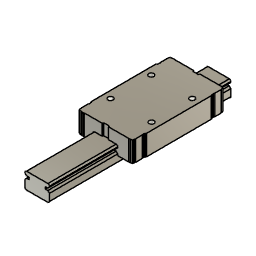
Wózek_prowadnica (Autodesk Fusion 360 design; units mm, degrees)
Autodesk Fusion 360 part; units mm, degrees
sketch "Szkic2" plane through (0, 0, 0) normal (0, 0, 1) x (1, 0, 0)
  line L0 (0.5477, 0.4589) -> (0.7, 0.3)
  line L1 (0.7, 0.3) -> (1.5, 0.1)
  line L2 (1.5, 0.1) -> (2.2904, 0.0655)
  line L3 (2.2904, 0.0655) -> (12.1473, 0.0943)
  line L4 (12.1473, 0.0943) -> (12.2508, 0.226)
  line L5 (12.2508, 0.226) -> (12.2979, 0.6305)
  line L6 (12.2979, 0.6305) -> (14.9884, 0.6384)
  line L7 (14.9884, 0.6384) -> (15.1105, 0.1602)
  line L8 (15.1105, 0.1602) -> (15.2422, 0.0849)
  line L9 (15.2422, 0.0849) -> (23.9813, 0.0755)
  line L10 (23.9813, 0.0755) -> (24.1318, -0.0185)
  line L11 (24.1318, -0.0185) -> (24.8468, -0.0193)
  line L12 (24.8468, -0.0193) -> (25.1383, 0.0473)
  line L13 (25.1383, 0.0473) -> (25.477, 0.0285)
  line L14 (25.477, 0.0285) -> (25.9944, 0.132)
  line L15 (25.9944, 0.132) -> (26.5172, 0.2365)
  line L16 (26.5172, 0.2365) -> (26.7093, 0.386)
  line L17 (26.7093, 0.386) -> (26.7658, 1.1103)
  line L18 (26.7658, 1.1103) -> (26.7846, 1.3737)
  line L19 (26.7846, 1.3737) -> (26.7093, 1.4583)
  line L20 (26.7093, 1.4583) -> (26.7991, 1.5382)
  line L21 (26.7991, 1.5382) -> (26.7991, 3.8)
  line L22 (26.7991, 3.8) -> (26.7752, 5.033)
  line L23 (26.7752, 5.033) -> (26.6905, 5.2399)
  line L24 (26.6905, 5.2399) -> (26.5964, 5.3905)
  line L25 (26.5964, 5.3905) -> (26.7469, 5.7009)
  line L26 (26.7469, 5.7009) -> (26.7187, 6.3217)
  line L27 (26.7187, 6.3217) -> (26.794, 6.4628)
  line L28 (26.794, 6.4628) -> (26.9182, 6.4584)
  line L29 (26.9182, 6.4584) -> (27.0302, 6.4999)
  line L30 (27.0302, 6.4999) -> (27.0298, 6.7378)
  line L31 (27.0298, 6.7378) -> (26.9182, 38.6182)
  line L32 (26.9182, 38.6182) -> (26.7385, 38.7234)
  line L33 (26.7385, 38.7234) -> (26.4901, 38.7638)
  line L34 (26.4901, 38.7638) -> (26.4901, 39.5761)
  line L35 (26.4901, 39.5761) -> (26.4001, 39.7061)
  line L36 (26.4001, 39.7061) -> (26.3026, 39.7711)
  line L37 (26.3026, 39.7711) -> (26.4526, 40.0485)
  line L38 (26.4526, 40.0485) -> (26.4776, 40.3735)
  line L39 (26.4776, 40.3735) -> (26.4951, 41.2983)
  line L40 (26.4951, 41.2983) -> (26.4968, 42.3691)
  line L41 (26.4968, 42.3691) -> (26.5013, 43.3724)
  line L42 (26.5013, 43.3724) -> (26.4887, 43.8502)
  line L43 (26.4887, 43.8502) -> (26.3606, 44.6632)
  line L44 (26.3606, 44.6632) -> (26.2, 44.8)
  line L45 (26.2, 44.8) -> (24.8739, 44.975)
  line L46 (24.8739, 44.975) -> (23.8326, 45.0084)
  line L47 (23.8326, 45.0084) -> (23.6823, 44.9193)
  line L48 (23.6823, 44.9193) -> (15, 44.9193)
  line L49 (15, 44.9193) -> (14.7953, 44.8414)
  line L50 (14.7953, 44.8414) -> (14.7, 44.4)
  line L51 (14.7, 44.4) -> (14.6673, 44.3458)
  line L52 (14.6673, 44.3458) -> (14, 44.3458)
  line L53 (14, 44.3458) -> (13.9156, 44.4237)
  line L54 (13.9156, 44.4237) -> (12.6, 44.4237)
  line L55 (12.6, 44.4237) -> (12.5736, 44.3458)
  line L56 (12.5736, 44.3458) -> (12.0446, 44.3402)
  line L57 (12.0446, 44.3402) -> (11.9444, 44.8024)
  line L58 (11.9444, 44.8024) -> (11.8, 44.9)
  line L59 (11.8, 44.9) -> (1.6, 44.9)
  line L60 (1.6, 44.9) -> (0.2956, 44.5713)
  line L61 (0.2956, 44.5713) -> (0.2, 43.7)
  line L62 (0.2, 43.7) -> (0.1898, 43.5829)
  line L63 (0.1898, 43.5829) -> (0.084, 43.5105)
  line L64 (0.084, 43.5105) -> (0.084, 40.4)
  line L65 (0.084, 40.4) -> (0.1938, 39.763)
  line L66 (0.1938, 39.763) -> (0.2522, 39.6776)
  line L67 (0.2522, 39.6776) -> (0.1741, 39.4042)
  line L68 (0.1741, 39.4042) -> (0.183, 38.7697)
  line L69 (0.183, 38.7697) -> (-0.0903, 38.7047)
  line L70 (-0.0903, 38.7047) -> (-0.1887, 38.5749)
  line L71 (-0.1887, 38.5749) -> (-0.0982, 38.3979)
  line L72 (-0.0982, 38.3979) -> (0, 6.6)
  line L73 (0, 6.6) -> (0.0316, 6.3256)
  line L74 (0.0316, 6.3256) -> (0.4567, 6.1485)
  line L75 (0.4567, 6.1485) -> (0.4583, 5.6223)
  line L76 (0.4583, 5.6223) -> (0.4876, 5.3675)
  line L77 (0.4876, 5.3675) -> (0.5427, 5.2629)
  line L78 (0.5427, 5.2629) -> (0.4061, 4.9289)
  line L79 (0.4061, 4.9289) -> (0.3657, 3.1467)
  line L80 (0.3657, 3.1467) -> (0.3282, 1.4919)
  line L81 (0.3282, 1.4919) -> (0.4744, 1.4321)
  line L82 (0.4744, 1.4321) -> (0.4219, 1.3038)
  line L83 (0.4219, 1.3038) -> (0.4716, 1.178)
  line L84 (0.4716, 1.178) -> (0.5322, 0.6214)
  line L85 (0.5322, 0.6214) -> (0.5477, 0.4589)
  circle A0 centre (23.448, 32.6514) radius 1.8526
  circle A1 centre (3.4408, 32.6002) radius 1.8346
  circle A2 centre (23.5356, 12.6463) radius 1.8379
  circle A3 centre (3.4921, 12.5855) radius 1.8455
  circle A4 centre (23.448, 32.6514) radius 1.5
  circle A5 centre (3.4408, 32.6002) radius 1.5
  circle A6 centre (23.5356, 12.6463) radius 1.5
  circle A7 centre (3.4921, 12.5855) radius 1.5
  dimension "d3" = 3
  dimension "d4" = 3
  dimension "d5" = 3
  dimension "d6" = 3
  constraint parallel L3 L6
  constraint parallel L9 L11
  constraint parallel L14 L15
  constraint perpendicular L19 L20
  constraint vertical L21
  constraint vertical L34
  constraint horizontal L48
  constraint parallel L48 L52
  constraint parallel L52 L54
  constraint horizontal L59
  constraint vertical L64
  constraint perpendicular L63 L66
  constraint parallel L72 L75
  constraint parallel L73 L76
  constraint parallel L79 L80
  constraint perpendicular L78 L81
  constraint perpendicular L81 L82
  constraint concentric A0 A4
  constraint concentric A1 A5
  constraint concentric A2 A6
  constraint concentric A3 A7
  measures "d3" diameter of A4
  measures "d4" diameter of A5
  measures "d5" diameter of A6
  measures "d6" diameter of A7
extrude "Wyciągnięcie proste1" add sketch "Szkic2" along normal blind 10 contours L0 L1 L2 L3 L4 L5 L6 L7 L8 L9 L10 L11 L12 L13 L14 L15 L16 L17 L18 L19 L20 L21 L22 L23 L24 L25 L26 L27 L28 L29 L30 L31 L32 L33 L34 L35 L36 L37 L38 L39 L40 L41 L42 L43 L44 L45 L46 L47 L48 L49 L50 L51 L52 L53 L54 L55 L56 L57 L58 L59 L60 L61 L62 L63 L64 L65 L66 L67 L68 L69 L70 L71 L72 L73 L74 L75 L76 L77 L78 L79 L80 L81 L82 L83 L84 L85 | A0 | A1 | A2 | A3 | A4 | A5 | A6 | A7 makes body 1
extrude "Wyciągnięcie proste2" cut sketch "Szkic2" along normal blind 6 contours A4 | A5 | A6 | A7 bodies 1
thread "Gwint1" "ISO Metric profile 3.0 M3x0.5 6H" major diameter 3.086 minor diameter 2.529 pitch 0.5 angle 60 resizes the face on face at (4.9902, 12.5108, 4) on bodies 1
thread "Gwint2" "ISO Metric profile 3.0 M3x0.5 6H" major diameter 3.086 minor diameter 2.529 pitch 0.5 angle 60 resizes the face on face at (25.0282, 12.7956, 4) on bodies 1
thread "Gwint3" "ISO Metric profile 3.0 M3x0.5 6H" major diameter 3.086 minor diameter 2.529 pitch 0.5 angle 60 resizes the face on face at (4.8504, 33.1132, 4) on bodies 1
thread "Gwint4" "ISO Metric profile 3.0 M3x0.5 6H" major diameter 3.086 minor diameter 2.529 pitch 0.5 angle 60 resizes the face on face at (24.8576, 33.1645, 4) on bodies 1
sketch "Szkic1" plane through (0, 0, 0) normal (0, 0, 1) x (1, 0, 0) in component "prowadnica_szyna v3"
  line L0 (0.75, 0) -> (11.25, 0)
  line L1 (11.25, 8) -> (0.75, 8)
  line L2 (6, 0) -> (6, 8)
  line L3 (12, 0.75) -> (12, 1.3964)
  line L4 (11.3964, 2) -> (10.5, 2)
  line L5 (10.5, 2) -> (10.5, 3)
  line L6 (10.5, 3) -> (11.3964, 3)
  line L7 (12, 0.75) -> (12, 1.3964)
  line L8 (12, 3.6036) -> (12, 7.25)
  line L9 (11.5732, 1.9268) -> (11.9268, 1.5732)
  line L10 (11.5732, 3.0732) -> (11.9268, 3.4268)
  arc A0 (11.5732, 1.9268) -> (11.3964, 2) centre (11.3964, 1.75) ccw
  arc A1 (12, 1.3964) -> (11.9268, 1.5732) centre (11.75, 1.3964) ccw
  arc A2 (11.3964, 3) -> (11.5732, 3.0732) centre (11.3964, 3.25) ccw
  arc A3 (11.9268, 3.4268) -> (12, 3.6036) centre (11.75, 3.6036) ccw
  arc A4 (11.25, 0) -> (12, 0.75) centre (11.25, 0.75) ccw
  arc A5 (12, 7.25) -> (11.25, 8) centre (11.25, 7.25) ccw
  line L11 (0.6036, 2) -> (1.5, 2)
  line L12 (0.4268, 1.9268) -> (0.0732, 1.5732)
  arc A6 (0, 0.75) -> (0.75, 0) centre (0.75, 0.75) ccw
  line L13 (0, 0.75) -> (0, 1.3964)
  line L14 (1.5, 2) -> (1.5, 3)
  line L15 (1.5, 3) -> (0.6036, 3)
  line L16 (0.4268, 3.0732) -> (0.0732, 3.4268)
  arc A7 (0.4268, 3.0732) -> (0.6036, 3) centre (0.6036, 3.25) ccw
  arc A8 (0, 3.6036) -> (0.0732, 3.4268) centre (0.25, 3.6036) ccw
  line L17 (0, 3.6036) -> (0, 7.25)
  arc A9 (0.75, 8) -> (0, 7.25) centre (0.75, 7.25) ccw
  arc A10 (0.0732, 1.5732) -> (0, 1.3964) centre (0.25, 1.3964) ccw
  arc A11 (0.6036, 2) -> (0.4268, 1.9268) centre (0.6036, 1.75) ccw
  line L18 (0, 7.25) -> (0, 3.6036)
  point P0 (12, 3)
  point P1 (11.5, 2)
  point P2 (12, 1.5)
  point P3 (11.5, 3)
  point P4 (12, 3.5)
  dimension "d3_1" = 1
  dimension "d6_1" = 0.5
  dimension "d7_1" = 0.5
  dimension "d8_1" = 0.25
  dimension "d9" = 0.75
  constraint horizontal L0
  constraint vertical L7
  constraint horizontal L1
  constraint vertical L18
  constraint perpendicular L4 L7
  constraint perpendicular L4 L5
  constraint coincident P0 L7
  constraint perpendicular L6 L7
  constraint collinear L7 L8
  constraint coincident P0 L6
  constraint coincident P0 L8
  constraint coincident P1 L9
  constraint coincident L4 P1
  constraint tangent L9 A0
  constraint tangent L4 A0
  constraint coincident P2 L9
  constraint coincident L3 P2
  constraint tangent L9 A1
  constraint tangent L3 A1
  constraint equal A0 A1
  constraint coincident P3 L10
  constraint coincident L6 P3
  constraint tangent L10 A2
  constraint tangent L6 A2
  constraint equal A0 A2
  constraint coincident P4 L10
  constraint coincident L8 P4
  constraint tangent L10 A3
  constraint tangent L8 A3
  constraint equal A0 A3
  constraint coincident L0 L2.start
  constraint tangent L0 A4
  constraint tangent L3 A4
  constraint coincident L1 L2.end
  constraint tangent L1 A5
  constraint tangent L8 A5
  constraint equal A4 A5
  constraint symmetric L2 L4.end L11.end
  constraint symmetric L2 L5.end L14.end
  constraint symmetric L2 L9.start L12.start
  constraint symmetric L2 L4.start L11.start
  constraint symmetric L2 A0 A11
  constraint symmetric L2 L9.end L12.end
  constraint symmetric L2 L3.end L13.end
  constraint symmetric L2 A1 A10
  constraint symmetric L2 L10.start L16.start
  constraint symmetric L2 L6.end L15.end
  constraint symmetric L2 A2 A7
  constraint symmetric L2 L10.end L16.end
  constraint symmetric L2 L8.start A8.start
  constraint symmetric L2 A3 A8
  constraint symmetric L2 L0.end L0.start
  constraint symmetric L2 L3.start A6.start
  constraint symmetric L2 A4 A6
  constraint symmetric L2 L1.start L1.end
  constraint symmetric L2 L8.end L17.end
  constraint symmetric L2 A5 A9
  measures "d3_1" distance of L4.end L5.end
  measures "d6_1" distance of P0 P3
  measures "d7_1" distance of P0 P4
  measures "d8_1" radius of A0
  measures "d9" radius of A4
extrude "Wyciągnięcie proste1'" add sketch "Szkic1" along normal blind 80 separate body makes body 2 in component "prowadnica_szyna v3"
sketch "Szkic2 (2)" plane through (0, 0, 80) normal (0, 0, 1) x (-1, 0, 0) in component "prowadnica_szyna v3"
  arc A0 (-11.5732, -1.9268) -> (-11.3964, -2) centre (-11.3964, -1.75) ccw
  line L0 (-11.3964, -2) -> (-10.5, -2)
  line L1 (-10.5, -2) -> (-10.5, -3)
  line L2 (-10.5, -3) -> (-11.3964, -3)
  arc A1 (-11.3964, -3) -> (-11.5732, -3.0732) centre (-11.3964, -3.25) ccw
  line L3 (-11.5732, -3.0732) -> (-11.9268, -3.4268)
  arc A2 (-11.9268, -3.4268) -> (-12, -3.6036) centre (-11.75, -3.6036) ccw
  line L4 (-12, -3.6036) -> (-12, -7.25)
  arc A3 (-12, -7.25) -> (-11.25, -8) centre (-11.25, -7.25) ccw
  line L5 (-11.25, -8) -> (-0.75, -8)
  arc A4 (-0.75, -8) -> (0, -7.25) centre (-0.75, -7.25) ccw
  line L6 (0, -7.25) -> (0, -3.6036)
  arc A5 (0, -3.6036) -> (-0.0732, -3.4268) centre (-0.25, -3.6036) ccw
  line L7 (-0.0732, -3.4268) -> (-0.4268, -3.0732)
  arc A6 (-0.4268, -3.0732) -> (-0.6036, -3) centre (-0.6036, -3.25) ccw
  line L8 (-0.6036, -3) -> (-1.5, -3)
  line L9 (-1.5, -3) -> (-1.5, -2)
  line L10 (-1.5, -2) -> (-0.6036, -2)
  arc A7 (-0.6036, -2) -> (-0.4268, -1.9268) centre (-0.6036, -1.75) ccw
  line L11 (-0.4268, -1.9268) -> (-0.0732, -1.5732)
  arc A8 (-0.0732, -1.5732) -> (0, -1.3964) centre (-0.25, -1.3964) ccw
  line L12 (0, -1.3964) -> (0, -0.75)
  arc A9 (0, -0.75) -> (-0.75, 0) centre (-0.75, -0.75) ccw
  line L13 (-0.75, 0) -> (-11.25, 0)
  arc A10 (-11.25, 0) -> (-12, -0.75) centre (-11.25, -0.75) ccw
  line L14 (-12, -0.75) -> (-12, -1.3964)
  arc A11 (-12, -1.3964) -> (-11.9268, -1.5732) centre (-11.75, -1.3964) ccw
  line L15 (-11.9268, -1.5732) -> (-11.5732, -1.9268)
  line L16 (0, -3.6036) -> (-2, -3.6036)
  line L17 (-2, -3.6036) -> (-2, -1.6787)
  line L18 (-1.5, -2) -> (-2, -2)
  line L19 (-1.5, -3) -> (-2, -3)
  line L20 (-6, 0) -> (-6, -8.8189)
  line L21 (-10.5, -3) -> (-10, -3)
  line L22 (-10.5, -2) -> (-10, -2)
  line L23 (-10, -3.6036) -> (-10, -1.6787)
  constraint coincident L6.end A5.start
  constraint perpendicular L6 L16
  constraint perpendicular L10 L17
  constraint coincident L9.end L10.start
  constraint coincident L17 L18.end
  constraint perpendicular L17 L18
  constraint coincident L8.end L9.start
  constraint coincident L17 L19.end
  constraint perpendicular L17 L19
  constraint midpoint L13 L20.start
  constraint perpendicular L13 L20
  constraint symmetric L16.end L20 L23.start
  constraint symmetric L17.end L20 L23.end
  constraint symmetric L9.end L20 L0.end
  constraint symmetric L18.end L20 L22.end
  constraint symmetric L8.end L20 L1.end
  constraint symmetric L19.end L20 L21.end
extrude "Wyciągnięcie proste2'" cut sketch "Szkic2 (2)" against normal blind 104 contours L1 L21 L22 L23 | L9 L17 L18 L19 bodies 2 in component "prowadnica_szyna v3"
sketch "Szkic3" plane through (0, 0, 80) normal (0, 0, 1) x (-1, 0, 0) in component "prowadnica_szyna v3"
  line L0 (-10, -3) -> (-11.3964, -3)
  arc A0 (-11.3964, -3) -> (-11.5732, -3.0732) centre (-11.3964, -3.25) ccw
  line L1 (-11.5732, -3.0732) -> (-11.9268, -3.4268)
  arc A1 (-11.9268, -3.4268) -> (-12, -3.6036) centre (-11.75, -3.6036) ccw
  line L2 (-12, -3.6036) -> (-12, -7.25)
  arc A2 (-12, -7.25) -> (-11.25, -8) centre (-11.25, -7.25) ccw
  line L3 (-11.25, -8) -> (-0.75, -8)
  arc A3 (-0.75, -8) -> (0, -7.25) centre (-0.75, -7.25) ccw
  line L4 (0, -7.25) -> (0, -3.6036)
  arc A4 (0, -3.6036) -> (-0.0732, -3.4268) centre (-0.25, -3.6036) ccw
  line L5 (-0.0732, -3.4268) -> (-0.4268, -3.0732)
  arc A5 (-0.4268, -3.0732) -> (-0.6036, -3) centre (-0.6036, -3.25) ccw
  line L6 (-0.6036, -3) -> (-2, -3)
  line L7 (-2, -3) -> (-2, -2)
  line L8 (-2, -2) -> (-0.6036, -2)
  arc A6 (-0.6036, -2) -> (-0.4268, -1.9268) centre (-0.6036, -1.75) ccw
  line L9 (-0.4268, -1.9268) -> (-0.0732, -1.5732)
  arc A7 (-0.0732, -1.5732) -> (0, -1.3964) centre (-0.25, -1.3964) ccw
  line L10 (0, -1.3964) -> (0, -0.75)
  arc A8 (0, -0.75) -> (-0.75, 0) centre (-0.75, -0.75) ccw
  line L11 (-0.75, 0) -> (-11.25, 0)
  arc A9 (-11.25, 0) -> (-12, -0.75) centre (-11.25, -0.75) ccw
  line L12 (-12, -0.75) -> (-12, -1.3964)
  arc A10 (-12, -1.3964) -> (-11.9268, -1.5732) centre (-11.75, -1.3964) ccw
  line L13 (-11.9268, -1.5732) -> (-11.5732, -1.9268)
  arc A11 (-11.5732, -1.9268) -> (-11.3964, -2) centre (-11.3964, -1.75) ccw
  line L14 (-11.3964, -2) -> (-10, -2)
  line L15 (-10, -2) -> (-10, -3)
  line L16 (0, -3) -> (-0.9, -3)
  line L17 (-0.9357, -2) -> (0, -2)
  line L18 (0, -2) -> (0, -1.2)
  line L19 (0, -3.8) -> (0, -4.6)
  line L20 (-0.8, -3) -> (-1.6, -3)
  line L21 (-0.8, -3) -> (0, -3.8)
  line L22 (-2, -2.5) -> (0.6, -2.5)
  line L23 (-0.8, -2) -> (0, -1.2)
  line L24 (-6, 0) -> (-6, -4)
  line L25 (-11.2, -3) -> (-12, -3.8)
  line L26 (-11.2, -2) -> (-12, -1.2)
  dimension "d14" = 0.8
  dimension "d15" = 0.8
  constraint coincident L6 L16.end
  constraint coincident L8 L17.start
  constraint perpendicular L7 L17
  constraint coincident L10 L18.end
  constraint perpendicular L17 L18
  constraint coincident L4 L19.end
  constraint perpendicular L16 L19
  constraint coincident L6 L20.end
  constraint coincident L16.start L20
  constraint coincident L16.start L19
  constraint midpoint L7 L22.start
  constraint perpendicular L7 L22
  constraint symmetric L20.start L22 L23.start
  constraint symmetric L19.start L22 L18.end
  constraint midpoint L11 L24.start
  constraint perpendicular L11 L24
  constraint symmetric L20.start L24 L25.start
  constraint symmetric L19.start L24 L25.end
  constraint symmetric L23.start L24 L26.start
  constraint symmetric L18.end L24 L26.end
  measures "d14" distance of L16.start L20.start
  measures "d15" distance of L16.start L19.start
extrude "Wyciągnięcie proste3" cut sketch "Szkic3" against normal blind 97 contours L0 A0 L1 A1 L2 L25 | L12 A10 L13 A11 L14 L26 | L4 A4 L5 A5 L6 L16 L21 | L8 A6 L9 A7 L10 L17 L18 L23 bodies 2 in component "prowadnica_szyna v3"
extrude "Wyciągnięcie proste4" cut 1 faces at (4.6667, 6.3333, 80) along direction (0, 0, -1) blind 25 on bodies 2 bodies 2 in component "prowadnica_szyna v3"
move_body "Przesuń1" bodies 1 to x (-0.999981, -0.006176, 0) y (-0.006176, 0.999981, 0) z (0, 0, -1) at (27.0406, 0.0835, 10)
sketch "Szkic3 (2)" plane through (0, -23.685, 0) normal (0, -1, 0) x (1, 0, 0)
  line L0 (0.8, 28.315) -> (0, 27.515)
  line L1 (0, 27.515) -> (0, 24.065)
  arc A0 (0, 24.065) -> (0.75, 23.315) centre (0.75, 24.065) ccw
  line L2 (0.75, 23.315) -> (11.25, 23.315)
  arc A1 (11.25, 23.315) -> (12, 24.065) centre (11.25, 24.065) ccw
  line L3 (12, 24.065) -> (12, 27.515)
  line L4 (12, 27.515) -> (11.2, 28.315)
  line L5 (11.2, 28.315) -> (10, 28.315)
  line L6 (10, 28.315) -> (10, 29.315)
  line L7 (10, 29.315) -> (11.2, 29.315)
  line L8 (11.2, 29.315) -> (12, 30.115)
  line L9 (12, 30.115) -> (12, 30.565)
  arc A2 (12, 30.565) -> (11.25, 31.315) centre (11.25, 30.565) ccw
  line L10 (11.25, 31.315) -> (0.75, 31.315)
  arc A3 (0.75, 31.315) -> (0, 30.565) centre (0.75, 30.565) ccw
  line L11 (0, 30.565) -> (0, 30.115)
  line L12 (0, 30.115) -> (0.8, 29.315)
  line L13 (0.8, 29.315) -> (2, 29.315)
  line L14 (2, 29.315) -> (2, 28.315)
  line L15 (2, 28.315) -> (0.8, 28.315)
  line L16 (6, 23.315) -> (6, 26.815)
  line L17 (0, 26.815) -> (12, 26.815)
  dimension "d20" = 3.5
  constraint midpoint L2 L16.start
  constraint perpendicular L2 L16
  constraint coincident L1 L17.start
  constraint coincident L3 L17.end
  constraint perpendicular L3 L17
  measures "d20" distance of L16.start L16.end
sketch "Szkic4" plane through (0, 0, 0) normal (0, 0, -1) x (1, 0, 0)
  line L0 (26.5046, -0.7016) -> (26.4901, -0.539)
  line L1 (26.4901, -0.539) -> (26.3388, -0.3792)
  line L2 (26.3388, -0.3792) -> (25.54, -0.1742)
  line L3 (25.54, -0.1742) -> (24.7499, -0.1349)
  line L4 (24.7499, -0.1349) -> (14.8929, -0.1028)
  line L5 (14.8929, -0.1028) -> (14.7886, -0.2339)
  line L6 (14.7886, -0.2339) -> (14.7391, -0.6381)
  line L7 (14.7391, -0.6381) -> (12.0486, -0.6293)
  line L8 (12.0486, -0.6293) -> (11.9294, -0.1504)
  line L9 (11.9294, -0.1504) -> (11.7982, -0.0743)
  line L10 (11.7982, -0.0743) -> (3.0593, -0.0109)
  line L11 (3.0593, -0.0109) -> (2.9094, 0.0841)
  line L12 (2.9094, 0.0841) -> (2.1945, 0.0893)
  line L13 (2.1945, 0.0893) -> (1.9025, 0.0244)
  line L14 (1.9025, 0.0244) -> (1.5639, 0.0454)
  line L15 (1.5639, 0.0454) -> (0.5225, -0.1563)
  line L16 (0.5225, -0.1563) -> (0.3294, -0.3045)
  line L17 (0.3294, -0.3045) -> (0.2685, -1.0285)
  line L18 (0.2685, -1.0285) -> (0.2481, -1.2917)
  line L19 (0.2481, -1.2917) -> (0.3228, -1.3769)
  line L20 (0.3228, -1.3769) -> (0.2326, -1.4561)
  line L21 (0.2326, -1.4561) -> (0.2186, -3.7179)
  line L22 (0.2186, -3.7179) -> (0.2349, -4.951)
  line L23 (0.2349, -4.951) -> (0.3183, -5.1585)
  line L24 (0.3183, -5.1585) -> (0.4114, -5.3096)
  line L25 (0.4114, -5.3096) -> (0.259, -5.6191)
  line L26 (0.259, -5.6191) -> (0.2834, -6.2401)
  line L27 (0.2834, -6.2401) -> (0.2073, -6.3807)
  line L28 (0.2073, -6.3807) -> (0.083, -6.3755)
  line L29 (0.083, -6.3755) -> (-0.0292, -6.4164)
  line L30 (-0.0292, -6.4164) -> (-0.0303, -6.6542)
  line L31 (-0.0303, -6.6542) -> (-0.1156, -38.5347)
  line L32 (-0.1156, -38.5347) -> (0.0635, -38.641)
  line L33 (0.0635, -38.641) -> (0.3117, -38.683)
  line L34 (0.3117, -38.683) -> (0.3066, -39.4953)
  line L35 (0.3066, -39.4953) -> (0.3958, -39.6258)
  line L36 (0.3958, -39.6258) -> (0.4929, -39.6914)
  line L37 (0.4929, -39.6914) -> (0.3412, -39.9679)
  line L38 (0.3412, -39.9679) -> (0.3142, -40.2927)
  line L39 (0.3142, -40.2927) -> (0.291, -41.2174)
  line L40 (0.291, -41.2174) -> (0.2826, -42.2881)
  line L41 (0.2826, -42.2881) -> (0.2719, -43.2914)
  line L42 (0.2719, -43.2914) -> (0.2816, -43.7693)
  line L43 (0.2816, -43.7693) -> (0.4047, -44.583)
  line L44 (0.4047, -44.583) -> (0.5644, -44.7208)
  line L45 (0.5644, -44.7208) -> (1.8895, -44.904)
  line L46 (1.8895, -44.904) -> (2.9305, -44.9439)
  line L47 (2.9305, -44.9439) -> (3.0814, -44.8557)
  line L48 (3.0814, -44.8557) -> (11.7635, -44.9093)
  line L49 (11.7635, -44.9093) -> (11.9686, -44.8326)
  line L50 (11.9686, -44.8326) -> (12.0667, -44.3919)
  line L51 (12.0667, -44.3919) -> (12.0998, -44.3379)
  line L52 (12.0998, -44.3379) -> (12.767, -44.342)
  line L53 (12.767, -44.342) -> (12.851, -44.4205)
  line L54 (12.851, -44.4205) -> (14.1665, -44.4286)
  line L55 (14.1665, -44.4286) -> (14.1934, -44.3508)
  line L56 (14.1934, -44.3508) -> (14.7224, -44.3485)
  line L57 (14.7224, -44.3485) -> (14.8198, -44.8113)
  line L58 (14.8198, -44.8113) -> (14.9636, -44.9098)
  line L59 (14.9636, -44.9098) -> (25.1634, -44.9728)
  line L60 (25.1634, -44.9728) -> (26.4698, -44.6521)
  line L61 (26.4698, -44.6521) -> (26.5707, -43.7814)
  line L62 (26.5707, -43.7814) -> (26.5817, -43.6644)
  line L63 (26.5817, -43.6644) -> (26.6879, -43.5927)
  line L64 (26.6879, -43.5927) -> (26.7071, -40.4822)
  line L65 (26.7071, -40.4822) -> (26.6013, -39.8446)
  line L66 (26.6013, -39.8446) -> (26.5433, -39.7587)
  line L67 (26.5433, -39.7587) -> (26.6232, -39.4859)
  line L68 (26.6232, -39.4859) -> (26.6182, -38.8513)
  line L69 (26.6182, -38.8513) -> (26.8919, -38.788)
  line L70 (26.8919, -38.788) -> (26.991, -38.6589)
  line L71 (26.991, -38.6589) -> (26.9017, -38.4813)
  line L72 (26.9017, -38.4813) -> (26.9999, -6.6834)
  line L73 (26.9999, -6.6834) -> (26.97, -6.4088)
  line L74 (26.97, -6.4088) -> (26.546, -6.2291)
  line L75 (26.546, -6.2291) -> (26.5476, -5.7029)
  line L76 (26.5476, -5.7029) -> (26.5199, -5.4479)
  line L77 (26.5199, -5.4479) -> (26.4654, -5.3429)
  line L78 (26.4654, -5.3429) -> (26.6041, -5.0098)
  line L79 (26.6041, -5.0098) -> (26.7032, -1.5734)
  line L80 (26.7032, -1.5734) -> (26.5574, -1.5127)
  line L81 (26.5574, -1.5127) -> (26.6107, -1.3847)
  line L82 (26.6107, -1.3847) -> (26.5617, -1.2586)
  line L83 (26.5617, -1.2586) -> (26.5046, -0.7016)
  line L84 (26.9508, -22.5823) -> (-0.0729, -22.5945)
  line L85 (13.4389, -22.5884) -> (13.3939, -0.6337)
  constraint midpoint L72 L84.start
  constraint midpoint L31 L84.end
  constraint midpoint L84 L85.start
  constraint midpoint L7 L85.end
extrude "Wyciągnięcie proste5" add 1 faces at (4.6667, 6.3333, 55) along direction (0, 0, 1) blind 34 on bodies 2 bodies 2 in component "prowadnica_szyna v3"
copy_body "Kopiuj-wklej bryły1" bodies 2 body 2 seen with x (-1, 0, 0) y (0, 0, -1) z (0, -1, 0) at (19.3939, 55.6337, 4.5) makes body 3
move_body "Przesuń2" bodies 3 to x (1, 0, 0) y (0, 1, 0) z (0, 0, 1) at (0, 0, 0)
combine "Kombinacja1" operation cut target body 1 tool bodies 2 body 2 seen with x (-1, 0, 0) y (0, 0, -1) z (0, -1, 0) at (19.3939, 55.6337, 4.5)
component "prowadnica_szyna v3" placed x (-1, 0, 0) y (0, 0, -1) z (0, -1, 0) at (19.3939, 55.6337, 4.5)
equation "d7_1 = d6_1"
equation "d15 = d14"
